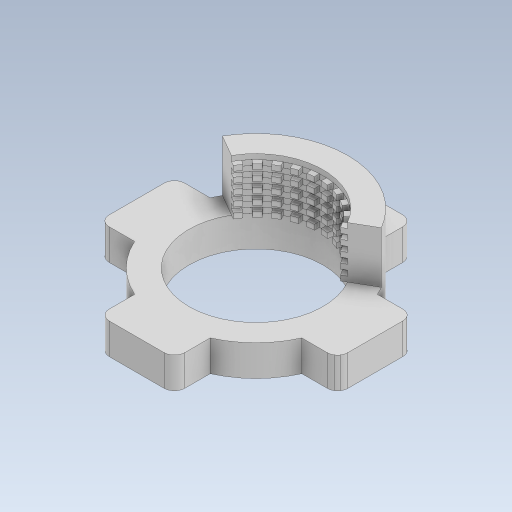
# Autodesk Inventor part: Plunger Cap
Saved by Autodesk Inventor 2023 (Build 270158000, 158)
## iProperties
Created: 2022-09-14
Part Number: Plunger Cap
Material: Generic
Document SubType Name: Modeling
Designer: Dave
Density: 1 g/cm^3
Appearance: Default
Author: Dave
Autodesk Inventor part; units mm, degrees
ref_plane "YZ Plane" through (0, 0, 0) normal (1, 0, 0) x (0, 1, 0)
ref_plane "XZ Plane" through (0, 0, 0) normal (0, 1, 0) x (-1, 0, 0)
sketch "Sketch1" plane through (0, 0, 0) normal (0, 1, 0) x (-1, 0, 0)
  arc A0 (16.223, 7.3) -> (7.325, 16.198) centre (0, -0.025) ccw
  line L0 (7.325, 16.198) -> (7.325, 21.125)
  arc A1 (7.325, 21.125) -> (7.025, 22.1786) centre (5.325, 21.125) ccw
  arc A2 (7.025, 22.1786) -> (6.3786, 22.825) centre (5.325, 21.125) ccw
  arc A3 (6.3786, 22.825) -> (5.325, 23.125) centre (5.325, 21.125) ccw
  line L1 (5.325, 23.125) -> (-5.325, 23.125)
  arc A4 (-5.325, 23.125) -> (-6.3786, 22.825) centre (-5.325, 21.125) ccw
  arc A5 (-6.3786, 22.825) -> (-7.025, 22.1786) centre (-5.325, 21.125) ccw
  arc A6 (-7.025, 22.1786) -> (-7.325, 21.125) centre (-5.325, 21.125) ccw
  line L2 (-7.325, 21.125) -> (-7.325, 16.198)
  arc A7 (-7.325, 16.198) -> (-16.223, 7.3) centre (0, -0.025) ccw
  line L3 (-16.223, 7.3) -> (-21.1473, 7.3)
  ellipse E0 centre (-21.2521, 5.3) end of major axis (-19.7618, 6.7142) minor radius 1.9496 (-21.1473, 7.3) -> (-22.218, 7) ccw
  ellipse E1 centre (-21.163, 5.3) end of major axis (-23.1657, 5.3) minor radius 2 (-22.218, 7) -> (-22.85, 6.3778) ccw
  ellipse E2 centre (-21.247, 5.3) end of major axis (-21.247, 7.3) minor radius 1.903 (-22.85, 6.3778) -> (-23.15, 5.3) ccw
  line L4 (-23.15, 5.3) -> (-23.15, -5.35)
  ellipse E3 centre (-21.247, -5.35) end of major axis (-21.247, -3.35) minor radius 1.903 (-23.15, -5.35) -> (-22.85, -6.4278) ccw
  ellipse E4 centre (-21.163, -5.35) end of major axis (-23.1657, -5.35) minor radius 2 (-22.85, -6.4278) -> (-22.218, -7.05) ccw
  ellipse E5 centre (-21.2521, -5.35) end of major axis (-22.7423, -3.9358) minor radius 1.9496 (-22.218, -7.05) -> (-21.1473, -7.35) ccw
  line L5 (-21.1473, -7.35) -> (-16.223, -7.35)
  arc A8 (-16.223, -7.35) -> (-7.325, -16.248) centre (0, -0.025) ccw
  line L6 (-7.325, -16.248) -> (-7.325, -21.175)
  line L7 (-7.025, -22.2286) -> (-7.025, -16.0531)
  arc A9 (-7.325, -21.175) -> (-7.025, -22.2286) centre (-5.325, -21.175) ccw
  arc A10 (-7.025, -22.2286) -> (-6.3786, -22.875) centre (-5.325, -21.175) ccw
  arc A11 (-6.3786, -22.875) -> (-5.325, -23.175) centre (-5.325, -21.175) ccw
  line L8 (-5.325, -23.175) -> (5.325, -23.175)
  line L9 (7.325, -21.175) -> (7.325, -16.248)
  arc A12 (7.025, -22.2286) -> (7.325, -21.175) centre (5.325, -21.175) ccw
  arc A13 (6.3786, -22.875) -> (7.025, -22.2286) centre (5.325, -21.175) ccw
  arc A14 (5.325, -23.175) -> (6.3786, -22.875) centre (5.325, -21.175) ccw
  arc A15 (7.325, -16.248) -> (16.223, -7.35) centre (0, -0.025) ccw
  line L10 (16.223, -7.35) -> (21.1473, -7.35)
  ellipse E6 centre (21.2521, -5.35) end of major axis (19.7618, -6.7642) minor radius 1.9496 (21.1473, -7.35) -> (22.218, -7.05) ccw
  ellipse E7 centre (21.163, -5.35) end of major axis (23.1657, -5.35) minor radius 2 (22.218, -7.05) -> (22.85, -6.4278) ccw
  ellipse E8 centre (21.247, -5.35) end of major axis (21.247, -7.35) minor radius 1.903 (22.85, -6.4278) -> (23.15, -5.35) ccw
  line L11 (23.15, -5.35) -> (23.15, 5.3)
  ellipse E9 centre (21.247, 5.3) end of major axis (21.247, 3.3) minor radius 1.903 (23.15, 5.3) -> (22.85, 6.3778) ccw
  ellipse E10 centre (21.163, 5.3) end of major axis (23.1657, 5.3) minor radius 2 (22.85, 6.3778) -> (22.218, 7) ccw
  ellipse E11 centre (21.2521, 5.3) end of major axis (22.7423, 3.8858) minor radius 1.9496 (22.218, 7) -> (21.1473, 7.3) ccw
  line L12 (21.1473, 7.3) -> (16.223, 7.3)
  circle A16 centre (0, -0.025) radius 13
  point P0 (0, 0)
  point P1 (0, 0)
  dimension "d0" = 26
  constraints: 32 point on circle, 26 end point, 17 centre point, 1 coincident, 1 vertical, 49 other
  measures "d0" diameter of A16
extrude "Extrusion1" add sketch "Sketch1" along normal blind 6
sketch "Sketch2" plane through (0, 6, 0) normal (0, 1, 0) x (1, 0, 0)
  circle A0 centre (0, 0.025) radius 13 projected
  line L0 (-13, 0.025) -> (-17.8, 0.025)
  arc A1 (17.8, 0.025) -> (-17.8, 0.025) centre (0, 0.025) ccw
  arc A2 (-7.325, 16.248) -> (-16.223, 7.35) centre (0, 0.025) ccw projected
  line L1 (13, 0.025) -> (17.8, 0.025)
  line L2 (-15.4153, 8.925) -> (-10.3923, 6.025)
  line L3 (10.3923, 6.025) -> (15.4153, 8.925)
  arc A3 (16.223, 7.35) -> (7.325, 16.248) centre (0, 0.025) ccw projected
  line L4 (0, 32.435) -> (0, -32.385) projected
  circle A4 centre (0, 0.025) radius 12
  point P0 (0, 0)
  point P1 (-11.2583, 6.525)
  point P2 (11.2583, 6.525)
  dimension "d3" = 120
  dimension "d6" = 1
  constraints: 10 point on circle, 8 end point, 2 centre point, 2 coincident, 2 horizontal, 2 horizontal alignment, 2 point on line, 1 concentric, 1 line through centre, 1 other
  measures "d3" angle of L3 L2
  measures "d6" radial gap between concentric circles of A0 A4
extrude "Extrusion2" add sketch "Sketch2" along normal blind 10 contours L3 A4 L4 A0 | A0 L4 A1 L3 | L4 A4 L2 A0 | A0 L2 A1 L4 picked at (10.4372, 7.0912) picked at (-10.4372, 7.0912)
sketch "Sketch3" plane through (0, 16, 0) normal (0, 1, 0) x (1, 0, 0)
  arc A0 (10.3923, 6.025) -> (-10.3923, 6.025) centre (0, 0.025) ccw projected
  circle A1 centre (0, 0) radius 12.0125
  line L0 (-11.2583, 6.525) -> (-10.3923, 6.025) projected
  circle A2 centre (0, 0) radius 13.0125
  line L1 (-10.3923, 6.025) -> (-11.2583, 6.525)
  arc A3 (11.2583, 6.525) -> (-11.2583, 6.525) centre (0, 0.025) ccw projected
  line L2 (-9.6664, 7.1317) -> (-10.4722, 7.7239)
  line L3 (-8.8232, 8.1518) -> (-9.5589, 8.8291)
  line L4 (-7.8729, 9.0729) -> (-8.5297, 9.827)
  line L5 (-6.827, 9.8839) -> (-7.3968, 10.7057)
  line L6 (-5.6983, 10.575) -> (-6.1742, 11.4545)
  line L7 (-4.5004, 11.1377) -> (-4.8767, 12.0642)
  line L8 (-3.2478, 11.5651) -> (-3.5199, 12.5274)
  line L9 (-1.9558, 11.8522) -> (-2.1204, 12.8386)
  line L10 (-0.6401, 11.9955) -> (-0.6952, 12.9939)
  line L11 (0.6834, 11.9931) -> (0.7384, 12.9915)
  line L12 (1.9985, 11.8451) -> (2.1631, 12.8315)
  line L13 (3.2895, 11.5534) -> (3.5616, 12.5156)
  line L14 (4.5405, 11.1214) -> (4.9168, 12.0479)
  line L15 (5.7364, 10.5544) -> (6.2123, 11.4338)
  line L16 (6.8626, 9.8593) -> (7.4324, 10.681)
  line L17 (7.9056, 9.0445) -> (8.5623, 9.7986)
  line L18 (8.8525, 8.1199) -> (9.5883, 8.7972)
  line L19 (9.6921, 7.0968) -> (10.4978, 7.689)
  line L20 (10.414, 5.9875) -> (11.28, 6.4875)
  point P0 (0.0028, 0.0248)
  point P1 (0.0055, 0.0244)
  point P2 (0.0081, 0.0236)
  point P3 (0.0107, 0.0226)
  point P4 (0.0131, 0.0213)
  point P5 (0.0154, 0.0197)
  point P6 (0.0174, 0.0179)
  point P7 (0.0193, 0.0159)
  point P8 (0.0209, 0.0137)
  point P9 (0.0223, 0.0113)
  point P10 (0.0234, 0.0088)
  point P11 (0.0242, 0.0061)
  point P12 (0.0248, 0.0034)
  point P13 (0.025, 0.0007)
  point P14 (0.0249, -0.0021)
  point P15 (0.0245, -0.0048)
  point P16 (0.0239, -0.0075)
  point P17 (0.0229, -0.01)
  point P18 (0.0217, -0.0125)
  point P19 (9.6939, 7.0981)
  point P20 (8.8558, 8.1229)
  point P21 (7.9097, 9.0492)
  point P22 (6.8672, 9.8658)
  point P23 (5.7409, 10.5627)
  point P24 (4.5445, 11.1312)
  point P25 (3.2926, 11.5644)
  point P26 (2.0005, 11.8571)
  point P27 (0.684, 12.0055)
  point P28 (-0.6408, 12.0079)
  point P29 (-1.9578, 11.8642)
  point P30 (-3.251, 11.5762)
  point P31 (-4.5044, 11.1475)
  point P32 (-5.7028, 10.5833)
  point P33 (-6.8316, 9.8906)
  point P34 (-7.8771, 9.0777)
  point P35 (-8.8265, 8.1548)
  point P36 (-9.6683, 7.133)
  dimension "d9" = 120
  constraints: 40 end point, 3 point on circle, 2 coincident, 1 centre point, 80 other
extrude "Extrusion3" cut sketch "Sketch3" against normal blind 10 contours A0 L18 A2 L19 | A0 L16 A2 L17 | L2 A2 L3 A0 | A0 L14 A2 L15 | L4 A2 L5 A0 | A0 L12 A2 L13 | L6 A2 L7 A0 | A0 L10 A2 L11 | L8 A2 L9 A0
sketch "Sketch4" plane through (15.4153, 6, -8.925) normal (0.5, 0, 0.8660254) x (0.8660254, 0, -0.5)
  line L0 (-5.8, 10) -> (0, 10) projected
  line L1 (-5.8, 10) -> (-4.8, 10)
  line L2 (-5.8, 0) -> (-4.8, 0) projected
  line L3 (-5.8, 10) -> (-5.8, 0)
  line L4 (-5.8, 0) -> (-4.8, 0)
  line L5 (-5.498, 10) -> (-5.498, 0) projected
  line L6 (-4.8, 0) -> (-4.8, 10)
  line L7 (-5.8, 9) -> (-4.8, 9)
  line L8 (-5.8, 8) -> (-4.8, 8)
  line L9 (-5.8, 7) -> (-4.8, 7)
  line L10 (-5.8, 6) -> (-4.8, 6)
  line L11 (-5.8, 5) -> (-4.8, 5)
  line L12 (-5.8, 4) -> (-4.8, 4)
  line L13 (-5.8, 3) -> (-4.8, 3)
  line L14 (-5.8, 2) -> (-4.8, 2)
  line L15 (-5.8, 1) -> (-4.8, 1)
  line L16 (-17.8125, -9.2) -> (-17.8125, 13.2) projected
  line L17 (-7.5305, 10) -> (-6.7156, 10) projected
  line L18 (-5.8, 0) -> (-6.7852, 0)
  line L19 (-6.7852, 0) -> (-6.7852, 10)
  line L20 (-6.7852, 10) -> (-5.8, 10)
  line L21 (-5.8, 10) -> (-5.8, 0)
  point P0 (-17.8125, -6)
  point P1 (-4.8, 1)
  point P2 (-4.8, 2)
  point P3 (-5.8, 2)
  point P4 (-5.8, 1)
  point P5 (-4.8, 3)
  point P6 (-4.8, 4)
  point P7 (-5.8, 4)
  point P8 (-5.8, 3)
  point P9 (-4.8, 5)
  point P10 (-4.8, 6)
  point P11 (-5.8, 6)
  point P12 (-5.8, 5)
  point P13 (-4.8, 7)
  point P14 (-4.8, 8)
  point P15 (-5.8, 8)
  point P16 (-5.8, 7)
  point P17 (-4.8, 9)
  point P18 (-4.8, 10)
  point P19 (-5.8, 9)
  dimension "d16" = 1
  constraints: 34 end point, 3 equal length, 3 vertical, 2 horizontal, 1 perpendicular, 1 point on line, 27 other
  measures "d16" distance of L0.start L7.start
revolve "Revolution1" cut sketch "Sketch4" angle 360 about axis through (-0.0108, -10, -0.0188) along (0, -1, 0) contours L0 L5 L7 L3 | L3 L18 L19 L17 L20 | L0 L6 L7 L5 | L8 L5 L9 L3 | L8 L6 L9 L5 | L10 L5 L11 L3 | L10 L6 L11 L5 | L3 L14 L5 L15 | L12 L5 L13 L3 | L5 L14 L6 L15 | L12 L6 L13 L5
sketch "Sketch5" plane through (-5.325, 0, 23.125) normal (0, 0, 1) x (1, 0, 0)
  line L0 (21.548, 0) -> (12.65, 0) projected
  line L1 (-2, 6) -> (12.65, 6)
  line L2 (12.65, 6) -> (12.65, 0)
  line L3 (12.65, 0) -> (-2, 0)
  line L4 (-2, 0) -> (-2, 6)
  point P0 (5.325, 0)
  constraints: 8 end point, 2 parallel, 1 horizontal, 1 perpendicular
sketch "Sketch6" plane through (0, 6, 0) normal (0, 1, 0) x (1, 0, 0)
  line L0 (-7.325, -16.198) -> (-7.325, -73.125) projected
  line L1 (-7.325, -31.7772) -> (7.325, -31.7772)
  line L2 (7.325, -31.7772) -> (7.325, -37.7772)
  line L3 (7.325, -37.7772) -> (-7.325, -37.7772)
  line L4 (-7.325, -37.7772) -> (-7.325, -31.7772)
  line L5 (7.325, -73.125) -> (7.325, -16.198) projected
  circle A0 centre (0, 0) radius 17.7772
  point P0 (-7.325, -37.7772)
  dimension "d28" = 35.5544
  dimension "d26" = 6
  dimension "d27" = 31.7772
  constraints: 8 end point, 2 parallel, 1 coincident, 1 collinear, 1 horizontal, 1 perpendicular, 1 point on line, 3 other
  measures "d26" distance of L3.end L1.start
  measures "d27" distance from line of L1 point (0, 0)
sketch "Sketch7" plane through (-5.325, 0, 73.125) normal (0, 0, 1) x (1, 0, 0)
  line L0 (-30.1072, 6) -> (56.6584, 6)
  line L1 (56.6584, 6) -> (56.6584, -21.378)
  line L2 (56.6584, -21.378) -> (-30.1072, -21.378)
  line L3 (-30.1072, -21.378) -> (-30.1072, 6)
  point P0 (5.325, 0)
  dimension "d41" = 2
  dimension "d42" = 10
  dimension "d46" = 10
  dimension "d54" = 10
  constraints: 2 midpoint, 1 centre point, 1 horizontal alignment, 1 vertical alignment
sketch "Sketch18" plane through (0, 6, 0) normal (0, -1, 0) x (1, 0, 0)
  arc A0 (0.6844, -12.0111) -> (2.0013, -11.8615) centre (-0.0108, -0.0188) ccw projected
  line L0 (0.6844, -12.0111) -> (0.7384, -12.9915) projected
  arc A1 (-0.6952, -12.9939) -> (0.7384, -12.9915) centre (0, 0) ccw projected
  line L1 (-0.6952, -12.9939) -> (-0.6412, -12.0147) projected
  arc A2 (-1.9592, -11.8722) -> (-0.6412, -12.0147) centre (-0.0108, -0.0188) ccw projected
  line L2 (-1.9592, -11.8722) -> (-2.1204, -12.8386) projected
  arc A3 (-3.5199, -12.5274) -> (-2.1204, -12.8386) centre (0, 0) ccw projected
  line L3 (-3.5199, -12.5274) -> (-3.2535, -11.5853) projected
  arc A4 (-4.5084, -11.1575) -> (-3.2535, -11.5853) centre (-0.0108, -0.0188) ccw projected
  line L4 (-4.5084, -11.1575) -> (-4.8767, -12.0642) projected
  arc A5 (-6.1742, -11.4545) -> (-4.8767, -12.0642) centre (0, 0) ccw projected
  line L5 (-6.1742, -11.4545) -> (-5.7086, -10.594) projected
  arc A6 (-6.8393, -9.9017) -> (-5.7086, -10.594) centre (-0.0108, -0.0188) ccw projected
  line L6 (-6.8393, -9.9017) -> (-7.3968, -10.7057) projected
  arc A7 (-8.5297, -9.827) -> (-7.3968, -10.7057) centre (0, 0) ccw projected
  line L7 (-8.5297, -9.827) -> (-7.8869, -9.0889) projected
  arc A8 (-8.8384, -8.1658) -> (-7.8869, -9.0889) centre (-0.0108, -0.0188) ccw projected
  line L8 (-8.8384, -8.1658) -> (-9.5589, -8.8291) projected
  arc A9 (-10.4722, -7.7239) -> (-9.5589, -8.8291) centre (0, 0) ccw projected
  line L9 (-10.4722, -7.7239) -> (-9.6824, -7.1434) projected
  arc A10 (-10.4085, -6.0344) -> (-9.6824, -7.1434) centre (-0.0108, -0.0188) ccw projected
  line L10 (-10.4085, -6.0344) -> (-15.4153, -8.925) projected
  arc A11 (-15.4153, -8.925) -> (15.4153, -8.925) centre (0, -0.025) ccw projected
  line L11 (15.4153, -8.925) -> (10.3923, -6.025) projected
  arc A12 (9.6939, -7.0981) -> (10.3923, -6.025) centre (-0.0108, -0.0188) ccw projected
  line L12 (9.6939, -7.0981) -> (10.4978, -7.689) projected
  arc A13 (9.5883, -8.7972) -> (10.4978, -7.689) centre (0, 0) ccw projected
  line L13 (9.5883, -8.7972) -> (8.856, -8.1231) projected
  arc A14 (7.9101, -9.0497) -> (8.856, -8.1231) centre (-0.0108, -0.0188) ccw projected
  line L14 (7.9101, -9.0497) -> (8.5623, -9.7986) projected
  arc A15 (7.4324, -10.681) -> (8.5623, -9.7986) centre (0, 0) ccw projected
  line L15 (7.4324, -10.681) -> (6.8678, -9.8668) projected
  arc A16 (5.7417, -10.5643) -> (6.8678, -9.8668) centre (-0.0108, -0.0188) ccw projected
  line L16 (5.7417, -10.5643) -> (6.2123, -11.4338) projected
  arc A17 (4.9168, -12.0479) -> (6.2123, -11.4338) centre (0, 0) ccw projected
  line L17 (4.9168, -12.0479) -> (4.5455, -11.1336) projected
  arc A18 (3.2936, -11.5678) -> (4.5455, -11.1336) centre (-0.0108, -0.0188) ccw projected
  line L18 (3.2936, -11.5678) -> (3.5616, -12.5156) projected
  arc A19 (2.1631, -12.8315) -> (3.5616, -12.5156) centre (0, 0) ccw projected
  line L19 (2.1631, -12.8315) -> (2.0013, -11.8615) projected
  circle A20 centre (0, 0) radius 13.0125
  line L20 (-6.8206, -16.4664) -> (-4.6052, -11.1179)
  arc A21 (-6.8393, -9.9017) -> (-5.7086, -10.594) centre (-0.0108, -0.0188) ccw projected
  line L21 (6.8206, -16.4664) -> (4.602, -11.1103)
  line L22 (0, -27.3746) -> (0, 39.4728) projected
  line L23 (-1.9592, -11.8722) -> (-2.1204, -12.8386) projected
  circle A22 centre (-0.0108, -0.0188) radius 12.0125
  line L24 (-4.6052, -11.1179) -> (-4.6052, 12.1704)
  line L25 (4.6052, -11.1179) -> (4.6052, 12.1704)
  line L26 (-4.9713, 29.9232) -> (-12.5103, 3.5803)
  line L27 (4.6052, 12.1704) -> (4.9713, 29.9232)
  line L28 (4.9713, 29.9232) -> (12.5103, 3.5803)
  line L29 (-4.6052, 12.1704) -> (-4.9713, 29.9232)
  point P0 (-4.9797, -12.022)
  point P1 (-8.5297, -9.827)
  point P2 (-11.2583, -6.525)
  point P3 (4.9797, -12.022)
  point P4 (11.2583, -6.525)
  point P5 (9.5883, -8.7972)
  point P6 (7.4324, -10.681)
  point P7 (-4.6052, 11.0804)
  point P8 (4.6052, 11.0804)
  point P9 (-10.4085, -6.0344)
  point P10 (-8.8384, -8.1658)
  point P11 (-8.5297, -9.827)
  point P12 (-6.8393, -9.9017)
  point P13 (4.6052, 11.0714)
  point P14 (4.6052, -11.1089)
  point P15 (5.7417, -10.5643)
  point P16 (7.4324, -10.681)
  point P17 (7.9101, -9.0497)
  point P18 (9.5883, -8.7972)
  point P19 (9.6939, -7.0981)
  point P20 (12.5103, 3.5803)
  dimension "d87" = 45
  constraints: 2 end point, 2 point on line, 1 horizontal, 1 tangent
  measures "d87" angle of L20 L21
sketch "Sketch20" plane through (-0.0108, 16, -13.0313) normal (0, 0, 1) x (1, 0, 0)
  line L0 (0, 0) -> (-5.3869, 0) projected
  line L1 (5.4085, 0) -> (0, 0) projected
  line L2 (5.4085, 0) -> (5.4085, 8) projected
  line L3 (-5.3869, 8) -> (5.4085, 8) projected
  line L4 (-5.3869, 0) -> (-5.3869, 8) projected
  point P0 (0.0108, -16)
sketch "Sketch23" plane through (-5.3977, 24, 21) normal (0, 0, 1) x (1, 0, 0)
  line L0 (10.7954, 0) -> (10.7954, -8) projected
  line L1 (0, 0) -> (10.7954, 0) projected
  line L2 (0, -8) -> (0, 0) projected
  line L3 (10.7954, -8) -> (0, -8) projected
  point P0 (5.3977, -24)
sketch "Sketch24" plane through (-5.3977, 16, 29) normal (0, -1, 0) x (1, 0, 0)
  line L0 (10.3824, -41.0341) -> (10.7954, -42.0313) projected
  line L1 (10.7954, -42.0313) -> (10.7954, 0) projected
  line L2 (10.7954, 0) -> (0, 0) projected
  line L3 (0, -42.0313) -> (0, 0) projected
  line L4 (0, -42.0313) -> (0.4098, -41.0418) projected
  arc A0 (0.4098, -41.0418) -> (10.3824, -41.0341) centre (5.3869, -29.0188) ccw projected
  line L5 (10.3977, -8) -> (0.3977, -8) projected
  line L6 (0, -8) -> (10.7954, -8) projected
  line L7 (10.7954, -8) -> (0, -8)
  point P0 (5.3977, -29)
  constraints: 2 end point, 1 perpendicular, 1 point on line
body "Solid1"
